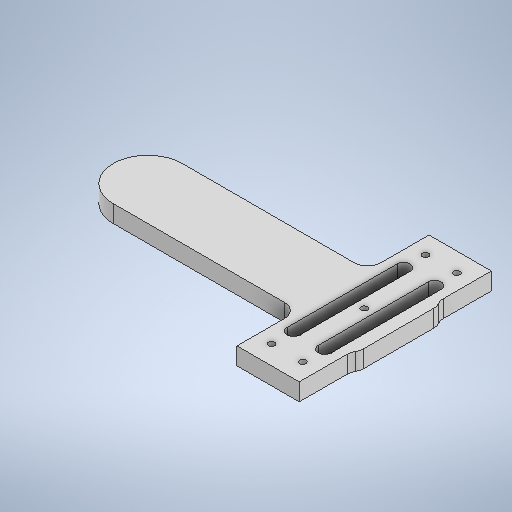
# Autodesk Inventor part: Chassis Front Spine
Saved by Autodesk Inventor 2025.2 (Build 292293000, 293)
## iProperties
Created: 2025-01-23
Part Number: Chassis Front Spine
Material: Generic
Document SubType Name: Modeling
Designer: Matt Tidd
Density: 1 g/cm^3
Appearance: Default
Author: Matt Tidd
Autodesk Inventor part; units mm, degrees
ref_plane "YZ Plane" through (0, 0, 0) normal (1, 0, 0) x (0, 1, 0)
ref_plane "XZ Plane" through (0, 0, 0) normal (0, 1, 0) x (-1, 0, 0)
ref_plane "XY Plane" through (0, 0, 0) normal (0, 0, 1) x (1, 0, 0)
sketch "Sketch13" plane through (0, 0, 0) normal (0, 1, 0) x (-1, 0, 0)
  line L0 (-18, 55.5) -> (18, 55.5)
  line L1 (18, 55.5) -> (18, -55.5)
  line L2 (18, -55.5) -> (-18, -55.5)
  line L3 (-18, -55.5) -> (-18, 55.5)
  line L4 (-18, 55.5) -> (18, -55.5) construction
  line L5 (18, 55.5) -> (-18, -55.5) construction
  line L6 (0, 55.5) -> (0, -55.5) construction
  line L7 (18, 0) -> (-18, 0) construction
  circle A0 centre (9, 44.5) radius 1.8
  circle A1 centre (-9, 44.5) radius 1.8
  circle A2 centre (9, -44.5) radius 1.8
  circle A3 centre (-9, -44.5) radius 1.8
  circle A4 centre (0, 0) radius 1.8
  line L8 (9, 31.75) -> (9, -31.75) construction
  line L9 (5.25, 31.75) -> (5.25, -31.75)
  line L10 (12.75, -31.75) -> (12.75, 31.75)
  arc A5 (12.75, 31.75) -> (5.25, 31.75) centre (9, 31.75) ccw
  arc A6 (5.25, -31.75) -> (12.75, -31.75) centre (9, -31.75) ccw
  line L11 (-5.25, 31.75) -> (-5.25, -31.75)
  line L12 (-12.75, -31.75) -> (-12.75, 31.75)
  arc A7 (-5.25, 31.75) -> (-12.75, 31.75) centre (-9, 31.75) ccw
  arc A8 (-12.75, -31.75) -> (-5.25, -31.75) centre (-9, -31.75) ccw
  arc A9 (18, 27.895) -> (19.0003, 24.0214) centre (26, 27.895) ccw
  line L13 (26, 27.895) -> (19.0003, 24.0214) construction
  line L14 (26, 27.895) -> (18, 27.895) construction
  arc A10 (19.0003, -24.0214) -> (18, -27.895) centre (26, -27.895) ccw
  line L15 (26, -27.895) -> (19.0003, -24.0214) construction
  line L16 (26, -27.895) -> (18, -27.895) construction
  line L17 (29.5178, 20.1478) -> (-2.9539, 20.1478) construction
  line L18 (19.0003, 24.0214) -> (12.0007, 20.1478) construction
  arc A11 (20.0007, 20.1478) -> (19.0003, 24.0214) centre (12.0007, 20.1478) ccw
  line L19 (12.0007, 20.1478) -> (20.0007, 20.1478) construction
  line L20 (12.0007, 20.1478) -> (19.0003, 24.0214) construction
  arc A12 (19.0003, -24.0214) -> (18, -27.895) centre (26, -27.895) ccw
  arc A13 (19.0003, -24.0214) -> (20.0007, -20.1478) centre (12.0007, -20.1478) ccw
  arc A14 (-19.0003, 24.0214) -> (-18, 27.895) centre (-26, 27.895) ccw
  arc A15 (-18, -27.895) -> (-19.0003, -24.0214) centre (-26, -27.895) ccw
  arc A16 (-19.0003, 24.0214) -> (-20.0007, 20.1478) centre (-12.0007, 20.1478) ccw
  arc A17 (-20.0007, -20.1478) -> (-19.0003, -24.0214) centre (-12.0007, -20.1478) ccw
  line L21 (20.0007, 20.1478) -> (20.0007, -20.1478)
  line L22 (-20.0007, 20.1478) -> (-20.0007, -20.1478)
  line L23 (18, 0) -> (26, 0) construction
  line L24 (20.0007, 0) -> (145.0007, 0) construction
  line L25 (145.0007, 0) -> (145.0007, -20) construction
  line L26 (145.0007, -20) -> (20.0007, -20) construction
  line L27 (20.0007, -20) -> (20.0007, 0) construction
  line L28 (145.0007, -20) -> (20.0007, -20)
  line L29 (20.0007, -20) -> (20.0007, 20)
  line L30 (20.0007, 20) -> (145.0007, 20)
  line L31 (145.0007, 20) -> (145.0007, -20)
  point P0 (9, 0)
  dimension "d93" = 36
  dimension "d94" = 111
  dimension "d95" = 3.6
  dimension "d96" = 3.6
  dimension "d97" = 7.5
  dimension "d98" = 28.96
  dimension "d99" = 28.96
  dimension "d100" = 8
  dimension "d101" = 28.96
  dimension "d102" = 8
  dimension "d103" = 125
  dimension "d104" = 20
  dimension "d105" = 125
  dimension "d106" = 40
  constraints: 66 end point, 28 symmetric about line, 26 point on circle, 18 centre point, 8 coincident, 8 midpoint, 8 parallel, 6 tangent, 5 perpendicular, 4 horizontal, 3 point on line, 1 vertical, 11 other
  measures "d93" distance of L1.end L2.end
  measures "d94" distance of L0.end L1.end
  measures "d95" diameter of A0
  measures "d96" diameter of A4
  measures "d97" diameter of A6
  measures "d98" angle of L14 L13
  measures "d99" angle of L15 L16
  measures "d100" distance of L18.start L18.end
  measures "d101" angle of L19 L20
  measures "d102" distance of L7.start L23.end
  measures "d103" distance of L25.end L26.end
  measures "d104" distance of L24.end L25.end
  measures "d105" distance of L29.end L30.end
  measures "d106" distance of L28.end L29.end
extrude "Extrusion11" add sketch "Sketch13" against normal blind 10
fillet "Fillet17" radius 8 2 edges at (-20.0007, -5, 20) (-20.0007, -5, -20)
fillet "Fillet18" radius 20 2 edges at (-145.0007, -5, 20) (-145.0007, -5, -20)
body "Solid2"
